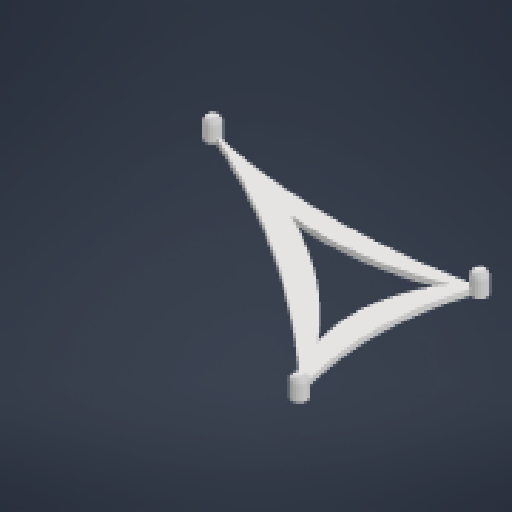
# Autodesk Inventor part: SiSpeedM1W_Holder
Saved by Autodesk Inventor 2024 (Build 280153000, 153)
## iProperties
Created: 2023-10-15
Part Number: SiSpeedM1W_Holder
Material: Generic
Document SubType Name: Modeling
Designer: Gurra
Density: 1 g/cm^3
Appearance: Default
Author: Gurra
Autodesk Inventor part; units mm, degrees
ref_plane "YZ Plane" through (0, 0, 0) normal (1, 0, 0) x (0, 1, 0)
ref_plane "XZ Plane" through (0, 0, 0) normal (0, 1, 0) x (-1, 0, 0)
ref_plane "XY Plane" through (0, 0, 0) normal (0, 0, 1) x (1, 0, 0)
sketch "Sketch1" plane through (0, 0, 0) normal (0, 1, 0) x (-1, 0, 0)
  circle A0 centre (48.4487, 3.6688) radius 1.25
  circle A1 centre (3.1987, 3.6688) radius 1.25
  circle A2 centre (3.1987, 34.2688) radius 1.25
  circle A3 centre (3.1987, 34.2688) radius 1.5
  circle A4 centre (3.1987, 3.6688) radius 1.5
  circle A5 centre (48.4487, 3.6688) radius 1.5
  arc A6 (4.6987, 34.2688) -> (48.4487, 5.1688) centre (117.9005, 157.023) ccw
  arc A7 (1.9487, 4.498) -> (1.9487, 33.4397) centre (-38.6824, 18.9688) ccw
  arc A8 (47.6195, 2.4188) -> (4.0278, 2.4188) centre (25.8237, -82.5805) ccw
  arc A9 (44.6935, 5.1688) -> (4.4426, 5.1664) centre (24.5711, -46.018) ccw
  arc A10 (4.4487, 31.9374) -> (44.6935, 5.1688) centre (72.5844, 90.7381) ccw
  arc A11 (4.4426, 5.1664) -> (4.4487, 31.9374) centre (-24.6203, 18.5585) ccw
  arc A12 (34.7326, 8.0352) -> (34.9553, 8.982) centre (35.5811, 8.3352) ccw
  arc A13 (5.0406, 6.549) -> (6.107, 5.7901) centre (5.6642, 6.2965) ccw
  arc A14 (6.7488, 29.373) -> (5.655, 28.9223) centre (6.2157, 29.1142) ccw
  point P0 (0, 0)
  point P1 (36.4803, 8.2972)
  point P2 (36.246, 7.7286)
  point P3 (5.6474, 5.624)
  dimension "d2" = 2.5
  dimension "d3" = 2.5
  dimension "d4" = 2.5
  dimension "d5" = 42.75
  dimension "d6" = 28.1
  dimension "d10" = 3
  dimension "d11" = 3
  dimension "d12" = 3
  dimension "d15" = 55
  dimension "d16" = 90
  dimension "d17" = 32
  constraints: 30 point on circle, 15 centre point, 3 coincident, 2 tangent
  measures "d2" diameter of A0
  measures "d3" diameter of A1
  measures "d4" diameter of A2
  measures "d10" diameter of A3
  measures "d11" diameter of A4
  measures "d12" diameter of A5
  measures "d15" radius of A9
  measures "d16" radius of A10
  measures "d17" radius of A11
extrude "Extrusion1" add sketch "Sketch1" along normal blind 2.5 contours A0 | A1 | A2 | A3 | A6 A5 A8 A4 A7 A3 | A5 | A4 | A9 A10 | A9 A12 | A13 A9 | A12 A10 A9 | A9 A11 A13 | A10 A12 | A11 A10 A14
sketch "Sketch2" plane through (0, 2.5, 0) normal (0, 1, 0) x (1, 0, 0)
  arc A0 (-4.6987, -34.2688) -> (-1.9487, -33.4397) centre (-3.1987, -34.2688) ccw projected
  circle A1 centre (-3.1987, -34.2688) radius 1.25
  arc A2 (-1.9487, -4.498) -> (-4.0278, -2.4188) centre (-3.1987, -3.6688) ccw projected
  circle A3 centre (-3.1987, -3.6688) radius 1.25
  arc A4 (-47.6195, -2.4188) -> (-48.4487, -5.1688) centre (-48.4487, -3.6688) ccw projected
  circle A5 centre (-48.4487, -3.6688) radius 1.25
  point P0 (0, 0)
  dimension "d20" = 2.5
  dimension "d21" = 2.5
  dimension "d22" = 2.5
  constraints: 3 centre point, 3 coincident
  measures "d20" diameter of A1
  measures "d21" diameter of A3
  measures "d22" diameter of A5
extrude "Extrusion2" add sketch "Sketch2" along normal blind 2.5
fillet "Fillet1" radius 1 3 edges at (-4.4487, 5, 34.2688) (-4.4487, 5, 3.6688) (-49.6987, 5, 3.6688)
body "Solid1"
